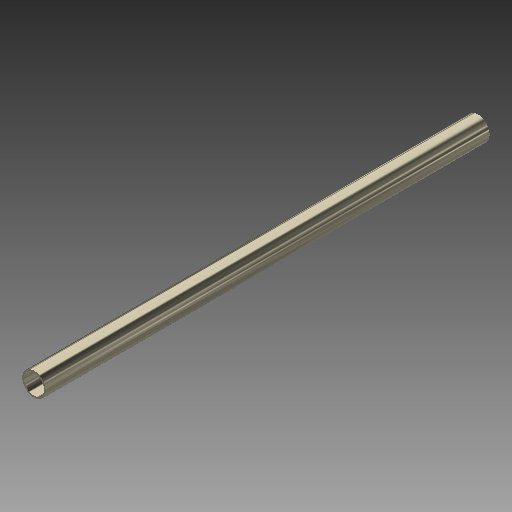
# Autodesk Inventor part: 202-05
Saved by Autodesk Inventor 2019 (Build 230136000, 136)
## iProperties
Company: Autodesk Inc.
Created: 2007-12-04
Part Number: 202-05
Document SubType Name: Modeling
Designer: Autodesk Inc.
Density: 7.85 g/cm^3
Mass: 285.294 g
Surface Area: 486.413 cm^2
Volume: 36.3431 cm^3
Material: Steel
Description: PIVOT BAR
Appearance: Nickel
Component Category: Back Component
Author: Inventor
Autodesk Inventor part; units mm, degrees
ref_plane "YZ Plane" through (0, 0, 0) normal (1, 0, 0) x (0, 1, 0)
ref_plane "XZ Plane" through (0, 0, 0) normal (0, 1, 0) x (-1, 0, 0)
ref_plane "XY Plane" through (0, 0, 0) normal (0, 0, 1) x (1, 0, 0)
sketch "Sketch1" plane through (0, 0, 0) normal (0, 0, 1) x (1, 0, 0)
  circle A0 centre (0, 0) radius 10.5
  circle A1 centre (0, 0) radius 9
  dimension "d0" = 18
  dimension "d1" = 21
  constraints: 2 centre point, 2 coincident
  measures "d0" diameter of A1
  measures "d1" diameter of A0
extrude "Extrusion1" add sketch "Sketch1" along normal mid plane 395.5
body "Solid1"
